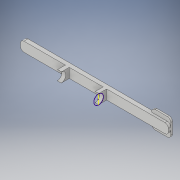
# Autodesk Inventor part: stweet
Saved by Autodesk Inventor 2018 (Build 220112000, 112)
## iProperties
Created: 2019-06-07
Part Number: stweet
Material: Generic
Document SubType Name: Modeling
Designer: 10043883
Density: 1 g/cm^3
Appearance: Default
Author: 10043883
Autodesk Inventor part; units mm, degrees
ref_plane "YZ Plane" through (0, 0, 0) normal (1, 0, 0) x (0, 1, 0)
ref_plane "XZ Plane" through (0, 0, 0) normal (0, 1, 0) x (-1, 0, 0)
ref_plane "XY Plane" through (0, 0, 0) normal (0, 0, 1) x (1, 0, 0)
sketch "Sketch1" plane through (0, 0, 0) normal (0, 0, 1) x (1, 0, 0)
  point P0 (0, 0)
sketch "Sketch2" plane through (0, 0, 0) normal (0, 0, 1) x (1, 0, 0)
  line L0 (0, 0) -> (137.16, 0)
  line L1 (137.16, 0) -> (137.16, 8.89)
  line L2 (137.16, 8.89) -> (0, 8.89)
  line L3 (0, 8.89) -> (0, 0)
  dimension "d0" = 137.16
  dimension "d3" = 8.89
  constraints: 8 end point, 2 parallel, 1 horizontal, 1 perpendicular
  measures "d0" distance of L2.end L1.end
  measures "d3" distance of L2.end L0.start
extrude "Extrusion1" add sketch "Sketch2" along normal blind 3.81
sketch "Sketch3" plane through (0, 8.89, 0) normal (0, 1, 0) x (1, 0, 0)
  line L0 (137.16, 0) -> (137.16, -3.81) projected
  line L1 (137.16, 0) -> (119.5015, 0)
  line L2 (119.5015, 0) -> (119.5015, -1.6003)
  line L3 (119.5015, -1.6003) -> (137.16, -1.6003)
  line L4 (137.16, -1.6003) -> (137.16, 0)
  point P0 (0, 0)
  constraints: 8 end point, 2 parallel, 1 horizontal, 1 perpendicular
extrude "Extrusion2" add sketch "Sketch3" along normal blind 3.81
sketch "Sketch4" plane through (0, 0, 0) normal (0, -1, 0) x (1, 0, 0)
  line L0 (0, 0) -> (137.16, 0) projected
  line L1 (119.5015, 1.6003) -> (137.16, 1.6003) projected
  line L2 (137.16, 0) -> (119.5015, 0)
  line L3 (119.5015, 0) -> (119.5015, 1.6003)
  line L4 (119.5015, 1.6003) -> (137.16, 1.6003)
  line L5 (137.16, 1.6003) -> (137.16, 0)
  constraints: 8 end point, 2 parallel, 1 horizontal, 1 perpendicular
extrude "Extrusion3" add sketch "Sketch4" along normal blind 3.81
sketch "Sketch6" plane through (0, 0, 3.81) normal (0, 0, 1) x (1, 0, 0)
  line L0 (119.5015, 8.89) -> (0, 8.89) projected
  line L1 (0, 0) -> (119.5015, 0) projected
  line L2 (79.905, 8.89) -> (76.6366, 8.89)
  line L3 (76.6366, 8.89) -> (76.6366, 0)
  line L4 (76.6366, 0) -> (79.905, 0)
  line L5 (79.905, 0) -> (79.905, 8.89)
  dimension "d28" = 119.5015
  constraints: 8 end point, 2 parallel, 2 point on line, 1 horizontal, 1 perpendicular
  measures "d28" distance of L1.start L1.end
extrude "Extrusion5" add sketch "Sketch6" along normal blind 7.62
sketch "Sketch7" plane through (79.905, 0, 3.81) normal (1, 0, 0) x (0, 0, -1)
  line L0 (-7.62, 0) -> (-7.62, 8.89) projected
  circle A0 centre (-7.62, 4.445) radius 4.445
  point P0 (3.81, 0)
  constraints: 1 midpoint, 1 vertical alignment, 2 other
extrude "Extrusion6" cut sketch "Sketch7" against normal blind 12.7
sketch "Sketch8" plane through (0, 0, 3.81) normal (0, 0, 1) x (1, 0, 0)
  line L0 (0, 0) -> (119.5015, 0) projected
  line L1 (119.5015, 8.89) -> (0, 8.89) projected
  line L2 (45.2172, 0) -> (41.5862, 0)
  line L3 (41.5862, 0) -> (41.5862, 8.89)
  line L4 (41.5862, 8.89) -> (45.2172, 8.89)
  line L5 (45.2172, 8.89) -> (45.2172, 0)
  constraints: 8 end point, 2 parallel, 2 point on line, 1 horizontal, 1 perpendicular
extrude "Extrusion7" add sketch "Sketch8" along normal blind 12.7
fillet "Fillet3" radius 3.175 8 edges at (0, 0, 1.905) (0, 8.89, 1.905) (137.16, 0, 2.7052) (137.16, 8.89, 2.7052) (137.16, -3.81, 0.8002) (137.16, 12.7, 0.8002) (119.5015, -3.81, 0.8002) (119.5015, 12.7, 0.8002)
extrude "Extrusion8" cut sketch "Sketch7" against normal through all
sketch "Sketch9" plane through (41.5862, 0, 16.51) normal (-1, 0, 0) x (0, 0, 1)
  circle A0 centre (-1.585, 4.5756) radius 5.8334
  point P0 (-16.51, 0)
  constraints: 1 centre point
extrude "Extrusion9" cut sketch "Sketch9" against normal through all
body "Solid1"
